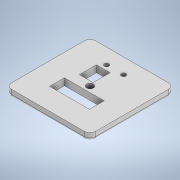
# Autodesk Inventor part: g2ExtruMountPlate
Saved by Autodesk Inventor 2020 (Build 240168000, 168)
## iProperties
Created: 2021-06-01
Part Number: g2ExtruMountPlate
Material: Generic
Document SubType Name: Modeling
Designer: PAB
Density: 1 g/cm^3
Appearance: Default
Author: PAB
Autodesk Inventor part; units mm, degrees
ref_plane "YZ Plane" through (0, 0, 0) normal (1, 0, 0) x (0, 1, 0)
ref_plane "XZ Plane" through (0, 0, 0) normal (0, 1, 0) x (-1, 0, 0)
ref_plane "XY Plane" through (0, 0, 0) normal (0, 0, 1) x (1, 0, 0)
sketch "Sketch1" plane through (0, 0, 0) normal (0, 1, 0) x (-1, 0, 0)
  line L0 (37, 37) -> (-37, 37)
  line L1 (-37, 37) -> (-37, -37)
  line L2 (-37, -37) -> (37, -37)
  line L3 (37, -37) -> (37, 37)
  point P0 (0, 0)
  dimension "d0" = 74
  dimension "d1" = 74
  constraints: 8 end point, 2 parallel, 1 horizontal, 1 perpendicular
  measures "d0" distance of L2.end L1.end
  measures "d1" distance of L1.end L0.end
extrude "Extrusion1" add sketch "Sketch1" along normal blind 6
fillet "Fillet1" radius 5 4 edges at (-37, 3, 37) (37, 3, 37) (37, 3, -37) (-37, 3, -37)
fillet "Fillet2" radius 2 8 edges at (35.5355, 0, 35.5355) (37, 0, 0) (35.5355, 0, -35.5355) (0, 0, -37) (-35.5355, 0, -35.5355) (-37, 0, 0) (-35.5355, 0, 35.5355) (0, 0, 37)
sketch "Sketch6" plane through (0, 6, 0) normal (0, 1, 0) x (1, 0, 0)
  circle A0 centre (0, 0) radius 3
  circle A1 centre (6.2, 23.4) radius 2
  circle A2 centre (-8.8, 23.4) radius 2
  line L0 (-1.3, 4) -> (-13.3, 4)
  line L1 (-13.3, 4) -> (-13.3, 19)
  line L2 (-13.3, 19) -> (-1.3, 19)
  line L3 (-1.3, 19) -> (-1.3, 4)
  line L4 (17.5, -5) -> (-17.5, -5)
  line L5 (-17.5, -5) -> (-17.5, -18)
  line L6 (-17.5, -18) -> (17.5, -18)
  line L7 (17.5, -18) -> (17.5, -5)
  dimension "d29" = 6
  dimension "d30" = 4
  dimension "d31" = 4
  dimension "d32" = 12
  dimension "d33" = 15
  dimension "d34" = 35
  dimension "d35" = 13
  constraints: 16 end point, 4 parallel, 3 centre point, 2 horizontal, 2 perpendicular, 1 coincident
  measures "d29" diameter of A0
  measures "d30" diameter of A1
  measures "d31" diameter of A2
  measures "d32" distance of L1.end L2.end
  measures "d33" distance of L0.end L1.end
  measures "d34" distance of L6.end L5.end
  measures "d35" distance of L5.end L4.end
extrude "Extrusion6" cut sketch "Sketch6" against normal blind 10
body "Solid1"
